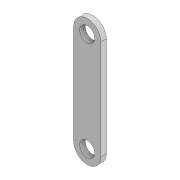
# Autodesk Inventor part: FirstPendulum
Saved by Autodesk Inventor 2020 (Build 240168000, 168)
## iProperties
Created: 2021-06-21
Part Number: FirstPendulum
Material: Generic
Document SubType Name: Modeling
Designer: Aidan Lee
Density: 1 g/cm^3
Appearance: Default
Author: Aidan Lee
Autodesk Inventor part; units mm, degrees
ref_plane "YZ Plane" through (0, 0, 0) normal (1, 0, 0) x (0, 1, 0)
ref_plane "XZ Plane" through (0, 0, 0) normal (0, 1, 0) x (-1, 0, 0)
ref_plane "XY Plane" through (0, 0, 0) normal (0, 0, 1) x (1, 0, 0)
sketch "Sketch1" plane through (0, 0, 0) normal (0, 0, 1) x (1, 0, 0)
  line L0 (0, 0) -> (220, 0) construction
  line L1 (220, 0) -> (220, 9) construction
  line L2 (220, 9) -> (0, 9) construction
  line L3 (0, 9) -> (0, 0) construction
  line L4 (0, 9) -> (90.94, 295.0593) construction
  line L5 (129.06, 295.0593) -> (220, 9) construction
  circle A0 centre (110, 289) radius 11 construction
  line L6 (96.1101, 281.616) -> (103.5522, 305.0259) construction
  arc A1 (129.06, 295.0593) -> (90.94, 295.0593) centre (110, 289) ccw construction
  line L7 (99, 275.5567) -> (99, 269.1274) construction
  line L8 (110, 289) -> (110, 143) construction
  line L9 (130, 289) -> (130, 143)
  line L10 (90, 143) -> (90, 289)
  arc A2 (130, 289) -> (90, 289) centre (110, 289) ccw
  arc A3 (90, 143) -> (130, 143) centre (110, 143) ccw
  line L11 (292.2692, 143) -> (292.2692, 247) construction
  line L12 (312.2692, 143) -> (312.2692, 247) construction
  line L13 (272.2692, 247) -> (272.2692, 143) construction
  arc A4 (272.2692, 143) -> (312.2692, 143) centre (292.2692, 143) ccw construction
  arc A5 (312.2692, 247) -> (272.2692, 247) centre (292.2692, 247) ccw construction
  arc A6 (90, 289) -> (130, 289) centre (110, 289) ccw construction
  line L14 (101.1908, 269) -> (118.8092, 269) construction
  line L15 (211.2941, 267) -> (373.2442, 267) construction
  line L16 (211.2941, 143) -> (373.2442, 143) construction
  line L17 (292.2692, 143) -> (292.2692, 39) construction
  line L18 (312.2692, 143) -> (312.2692, 39) construction
  line L19 (272.2692, 39) -> (272.2692, 143) construction
  arc A7 (312.2692, 143) -> (272.2692, 143) centre (292.2692, 143) ccw construction
  arc A8 (272.2692, 39) -> (312.2692, 39) centre (292.2692, 39) ccw construction
  line L20 (211.2941, 19) -> (373.2442, 19) construction
  circle A9 centre (110, 289) radius 11
  circle A10 centre (110, 143) radius 11
  point P0 (110, 0)
  point P1 (110, 216)
  point P2 (110, 309)
  point P3 (292.2692, 195)
  point P4 (110, 269)
  point P5 (110, 269)
  point P6 (292.2692, 267)
  dimension "d0" = 9
  dimension "d1" = 220
  dimension "d2" = 22
  dimension "d3" = 280
  dimension "d4" = 9
  dimension "d7" = 40
  dimension "d8" = 40
  dimension "pendgap" = 2
  dimension "abovethefloor" = 10
  dimension "d11" = 104
  dimension "d12" = 146
  dimension "d14" = 22
  constraints: 48 end point, 19 point on circle, 14 tangent, 11 centre point, 6 midpoint, 5 coincident, 5 parallel, 5 symmetric about line, 4 horizontal, 3 vertical, 2 vertical alignment, 1 concentric, 1 horizontal alignment, 1 perpendicular, 2 other
  measures "d0" distance of L2.end L0.start
  measures "d1" distance of L0.start L0.end
  measures "d2" diameter of A0
  measures "d3" distance from line of L2 A0.centre
  measures "d4" distance between parallel lines of L4 L6
  measures "d7" distance between parallel lines of L9 L10
  measures "d8" distance between parallel lines of L12 L13
  measures "pendgap" distance between parallel lines of L15 L14
  measures "abovethefloor" distance between parallel lines of L2 L20
  measures "d11" distance of L11.start L17.end
  measures "d12" distance of A0.centre L8.end
  measures "d14" diameter of A10
extrude "Extrusion2" add sketch "Sketch1" along normal blind 8
body "Solid2"
